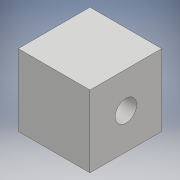
# Autodesk Inventor part: 01Cubo
Saved by Autodesk Inventor 2018 (Build 220112000, 112)
## iProperties
Created: 2020-06-22
Part Number: 01Cubo
Material: Generic
Document SubType Name: Modeling
Designer: Ivan
Density: 1 g/cm^3
Appearance: Default
Author: Ivan
Autodesk Inventor part; units mm, degrees
ref_plane "YZ Plane" through (0, 0, 0) normal (1, 0, 0) x (0, 1, 0)
ref_plane "XZ Plane" through (0, 0, 0) normal (0, 1, 0) x (-1, 0, 0)
ref_plane "XY Plane" through (0, 0, 0) normal (0, 0, 1) x (1, 0, 0)
sketch "Sketch1" plane through (0, 0, 0) normal (0, 0, 1) x (1, 0, 0)
  line L0 (0, 0) -> (10, 0)
  line L1 (-2, 0) -> (12, 0) construction
  line L2 (0, 0) -> (0, 10)
  line L3 (10, 0) -> (10, 10)
  line L4 (0, 10) -> (10, 10)
  dimension "d0" = 10
  dimension "d1" = 10
  dimension "d2" = 10
  constraints: 8 end point, 2 collinear, 1 parallel, 1 perpendicular
  measures "d0" distance of L0.start L0.end
  measures "d1" distance of L0.start L2.end
  measures "d2" distance of L0.end L3.end
extrude "Extrusion1" add sketch "Sketch1" along normal blind 10
sketch "Sketch2" plane through (10, 0, 0) normal (1, 0, 0) x (0, 0, -1)
  circle A0 centre (-5, 5) radius 1.5
  line L0 (-10, 0) -> (-10, 10) projected
  line L1 (0, 0) -> (-10, 0) projected
  point P0 (-10, 5)
  point P1 (-5, 0)
  dimension "d5" = 3
  constraints: 2 midpoint, 1 centre point, 1 horizontal alignment, 1 vertical alignment
  measures "d5" diameter of A0
extrude "Extrusion2" cut sketch "Sketch2" against normal up to surface (10 mm away)
equation "\"d1\" = d0"
equation "\"d2\" = d1"
body "Solid1"
